13af26b5-eefb-45c6-a7dd-1461c027063c (Autodesk Fusion 360 design; units mm, degrees)
Autodesk Fusion 360 part; units mm, degrees
sketch "Sketch2" plane through (0, 0, 0) normal (1, 0, 0) x (0, 1, 0)
  line L0 (0, 0) -> (19.05, 0) construction
  line L1 (38.6334, 0) -> (19.05, 0) construction
  circle A0 centre (28.8417, 0) radius 9.7917
  dimension "d1" = 19.05
  dimension "d2" = 38.6334
  constraint coincident L0.start origin
  constraint horizontal L0
  constraint parallel L0 L1
  constraint midpoint L1 A0.centre
  constraint coincident L1.start A0
  measures "d1" distance of L0.start L0.end
  measures "d2" distance of L0.start L1.start
revolve "Revolve4" add sketch "Sketch2" angle 360 about axis through (0, 0, 1.75) along (0, 0, 1) makes body 1
ref_plane "WorkPlane1" through (-38.6334, 0, 0) normal (1, 0, 0) x (0, 1, 0)
ref_plane "WorkPlane2" through (104.2416, 0, 0) normal (1, 0, 0) x (0, 1, 0)
ref_plane "WorkPlane3" through (40.7416, 0, 0) normal (1, 0, 0) x (0, 1, 0)
sketch "Sketch6" plane through (40.7416, 0, 0) normal (1, 0, 0) x (0, 1, 0)
  circle A0 centre (0, 0) radius 9.525
  dimension "d31" = 19.05
  constraint coincident A0.centre origin
  measures "d31" diameter of A0
extrude "Extrude1" add sketch "Sketch6" along normal up to surface (63.5 mm away) separate body makes body 2
ref_plane "WorkPlane4" through (28.8417, 0, 0) normal (1, 0, 0) x (0, 1, 0)
sketch "Sketch7" plane through (0, 0, 0) normal (0, 0, 1) x (1, 0, 0)
  line L0 (28.8417, 0.75) -> (28.8417, 21.75)
  line L1 (0, 0) -> (76.2, 0) construction
  line L2 (28.8417, 18.7283) -> (28.8417, -25.4) construction
  line L3 (28.8417, 0) -> (57.4167, 0)
  line L4 (57.4167, 0) -> (57.4167, 16.8776)
  line L5 (28.8417, 0) -> (28.8417, 9.525)
  line L6 (51.9955, 20.3301) -> (28.8417, 9.525)
  arc A0 (57.4167, 16.8776) -> (51.9955, 20.3301) centre (53.6067, 16.8776) ccw
  point P0 (57.4167, 22.86)
  dimension "d40" = 28.575
  dimension "d41" = 22.86
  dimension "d42" = 9.525
  dimension "d43" = 3.81
  constraint coincident L1.start origin
  constraint horizontal L1
  constraint coincident L0 L2.start
  constraint parallel L0 L2
  constraint coincident L2 L3.start
  constraint coincident L1 L3.start
  constraint perpendicular L2 L3
  constraint perpendicular L3 L4
  constraint perpendicular L3 L5
  constraint coincident P0 L4
  constraint coincident P0 L6
  constraint tangent L4 A0
  constraint tangent L6 A0
  measures "d40" distance of L3.start L3.end
  measures "d41" distance of L3.end P0
  measures "d42" distance of L3.start L5.end
  measures "d43" radius of A0
revolve "Revolve5" add sketch "Sketch7" angle 360 about axis through (0, 0, 0) along (1, 0, 0) bodies 1 2
thread "Thread2" "ANSI Unified Screw Threads 0.3125 5/16-18 UNC 3A" major diameter 7.8283 minor diameter 6.2586 pitch 1.4111 angle 60 modelled right hand crest width 0.2172 on face at (73.025, 9.4777, 0.9484) crest through (57.0639, 3.9141, 0) on bodies 1
fillet "Fillet2" radius 3.81 1 edges at (36.3437, -12.9998, -0.824) on bodies 1
equation "d27 = -d2"
equation "d28 = 5.625 in"
equation "d30 = -2.500 in"
equation "EyeInner = d1"
equation "EyeOuter = d2"
equation "ThreadDia = d31"
equation "TotalLength = d28"
equation "ShankLength = d30"
equation "d39 = d1 + ( ( d2 - d1 ) ) / 2"
equation "d40 = d31 * 1.5"
equation "d41 = d31 * 1.2"
equation "d42 = d31 / 2"
equation "d43 = d31 * 0.2"
equation "d45 = d31 * 0.2"
